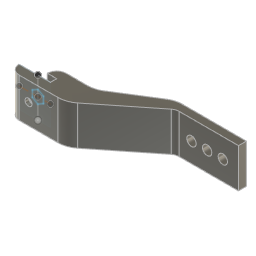
CR6_SE_CameraBedMount_WithNutExtended (Autodesk Fusion 360 design; units mm, degrees)
Autodesk Fusion 360 part; units mm, degrees
sketch "Sketch1" plane through (0, 0, 0) normal (0, 0, 1) x (1, 0, 0)
  line L0 (0, 0) -> (0, 6)
  line L1 (0, 6) -> (20, 6)
  line L2 (20, 6) -> (20, 10)
  line L3 (20, 10) -> (14, 10)
  line L4 (14, 16) -> (14, 10)
  line L5 (14, 16) -> (38, 16)
  line L6 (38, 16) -> (70, 36)
  line L7 (70, 36) -> (115, 36)
  line L8 (115, 36) -> (115, 31)
  line L9 (115, 31) -> (75, 31)
  line L10 (75, 31) -> (36, 0)
  line L11 (36, 0) -> (0, 0)
  dimension "d1" = 4
  dimension "d2" = 24
  dimension "d6" = 115
  dimension "d7" = 5
  dimension "d8" = 45
  dimension "d10" = 20
  dimension "d11" = 36
  dimension "d12" = 16
  dimension "d13" = 6
  dimension "d14" = 14
  dimension "d15" = 36
  dimension "d16" = 40
  constraint coincident L0.start L11.end
  constraint vertical L0
  constraint perpendicular L0 L1
  constraint perpendicular L1 L2
  constraint perpendicular L2 L3
  constraint perpendicular L3 L4
  constraint perpendicular L4 L5
  constraint perpendicular L4 L7
  constraint perpendicular L7 L8
  constraint perpendicular L8 L9
  constraint perpendicular L0 L11
  measures "d1" distance of L1.end L2.end
  measures "d2" distance of L4.start L5.end
  measures "d6" distance of L0 L8
  measures "d7" distance of L7.end L8.end
  measures "d8" distance of L6.end L7.end
  measures "d10" distance of L0.end L1.end
  measures "d11" distance of L10.end L0.start
  measures "d12" distance of L5 L11
  measures "d13" distance of L0.start L0.end
  measures "d14" distance of L0 L4
  measures "d15" distance of L7 L11
  measures "d16" distance of L8.end L9.end
extrude "Extrude1" add sketch "Sketch1" along normal blind 25
sketch "Sketch2" plane through (0, 6, 0) normal (0, 1, 0) x (-1, 0, 0)
  line L0 (-20, 0) -> (0, 0)
  line L1 (0, 0) -> (0, 25)
  line L2 (0, 25) -> (-20, 25)
  line L3 (-20, 25) -> (-20, 0)
  line L4 (0, 13) -> (-20, 13) construction
  line L5 (-12, 25) -> (-12, 0) construction
  line L6 (-8.5, 15.0207) -> (-12, 17.0415)
  line L7 (-12, 17.0415) -> (-15.5, 15.0207)
  line L8 (-15.5, 15.0207) -> (-15.5, 10.9793)
  line L9 (-15.5, 10.9793) -> (-12, 8.9585)
  line L10 (-12, 8.9585) -> (-8.5, 10.9793)
  line L11 (-8.5, 10.9793) -> (-8.5, 15.0207)
  point P0 (-12, 13)
  dimension "d19" = 12
  dimension "d20" = 3.5
  constraint coincident L1 L4.start
  constraint coincident L3 L4.end
  constraint perpendicular L3 L4
  constraint coincident L2 L5.start
  constraint perpendicular L4 L5
  constraint coincident L4 P0
  constraint coincident L5 P0
  measures "d19" distance of L1 L5
  measures "d20" distance of P0 L11
extrude "Extrude2" cut sketch "Sketch2" against normal blind 3.5 contours L6 L7 L8 L9 L10 L11
hole "Hole1" at (12, 6, 13) direction (0, -1, 0) diameter 4.5 end through all
sketch "Sketch3" plane through (0, 36, 0) normal (0, 1, 0) x (-1, 0, 0)
  line L0 (-115, 0) -> (-70, 0)
  line L1 (-70, 0) -> (-70, 25)
  line L2 (-70, 25) -> (-115, 25)
  line L3 (-115, 25) -> (-115, 0)
  line L4 (-115, 12.5) -> (-70, 12.5) construction
  line L5 (-105, 25) -> (-105, 0) construction
  point P0 (-105, 12.5)
  dimension "d26" = 10
  constraint midpoint L3 L4.start
  constraint midpoint L1 L4.end
  constraint coincident L2 L5.start
  constraint coincident L0 L5.end
  constraint perpendicular L0 L5
  constraint midpoint L5 P0
  measures "d26" distance of L3 L5
hole "Hole2" at (105, 36, 12.5) direction (0, -1, 0) diameter 6 depth 6.5 tip angle 118
pattern_linear "R-Pattern1" count 3 spacing 10 along (-1, 0, 0) of "Hole2"
fillet "Fillet1" radius 15 1 edges at (70, 36, 12.5)
fillet "Fillet1" radius 6 1 edges at (75, 31, 12.5)
fillet "Fillet2" radius 15 2 edges at (38, 16, 12.5) (36, 0, 12.5)
fillet "Fillet3" radius 6 1 edges at (14, 16, 12.5)
fillet "Fillet4" radius 6 1 edges at (0, 0, 12.5)
